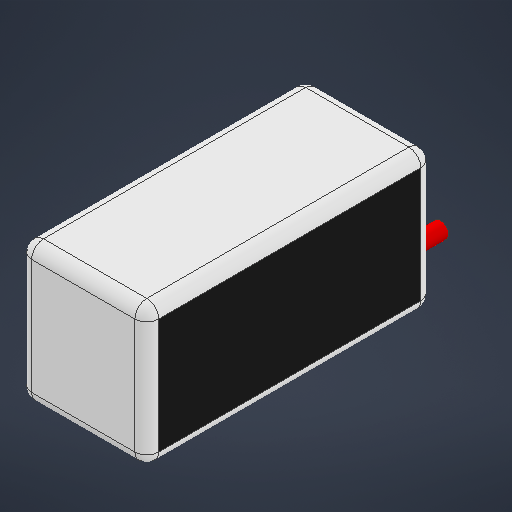
# Autodesk Inventor part: SLS Quantum 1300mAh 4S1P 14,8V 65C
Saved by Autodesk Inventor 2026.1 (Build 301233020, 233B)
## iProperties
Created: 2025-11-20
Part Number: SLS Quantum 1300mAh 4S1P 14,8V 65C
Material: Generic
Document SubType Name: Modeling
Designer: Bahaa
Density: 1 g/cm^3
Appearance: Default
Author: Bahaa
Autodesk Inventor part; units mm, degrees
ref_plane "YZ Plane" through (0, 0, 0) normal (1, 0, 0) x (0, 1, 0)
ref_plane "XZ Plane" through (0, 0, 0) normal (0, 1, 0) x (-1, 0, 0)
ref_plane "XY Plane" through (0, 0, 0) normal (0, 0, 1) x (1, 0, 0)
sketch "Sketch1" plane through (0, 0, 0) normal (0, 1, 0) x (-1, 0, 0)
  line L0 (16, 17.5) -> (-16, 17.5)
  line L1 (-16, 17.5) -> (-16, -17.5)
  line L2 (-16, -17.5) -> (16, -17.5)
  line L3 (16, -17.5) -> (16, 17.5)
  line L4 (16, 17.5) -> (-16, -17.5) construction
  line L5 (-16, 17.5) -> (16, -17.5) construction
  line L6 (0, -17.5) -> (0, -14.5) construction
  line L7 (0, -14.5) -> (3, -14.5) construction
  circle A0 centre (3, -14.5) radius 2
  circle A1 centre (-3, -14.5) radius 2
  point P0 (0, 0)
  dimension "d0" = 32
  dimension "d1" = 35
  dimension "d5" = 3
  dimension "d6" = 3
  dimension "d7" = 4
  constraints: 16 end point, 3 midpoint, 2 centre point, 2 horizontal, 2 parallel, 1 coincident, 1 perpendicular, 1 symmetric about line, 1 vertical, 1 other
  measures "d0" distance of L2.end L1.end
  measures "d1" distance of L1.end L0.end
  measures "d5" distance of L6.start L6.end
  measures "d6" distance of L6.end L7.end
  measures "d7" diameter of A0
extrude "Extrusion1" add sketch "Sketch1" along normal blind 72 contours L3 L2 L1 L0 | A0 | A1
extrude "Extrusion2" add sketch "Sketch1" along normal blind 15 from surface at 72 contours A0 | A1
fillet "Fillet1" radius 3 12 edges at (16, 36, 17.5) (16, 36, -17.5) (-16, 36, 17.5) (-16, 36, -17.5) (16, 72, 0) (0, 72, 17.5) (0, 72, -17.5) (-16, 72, 0) (16, 0, 0) (0, 0, 17.5) (-16, 0, 0) (0, 0, -17.5)
body "Solid1"
